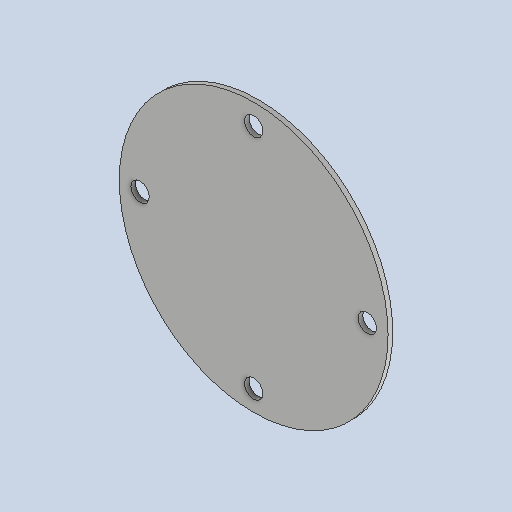
# Autodesk Inventor part: MSC 126 flange base tube
Saved by Autodesk Inventor 2025 (Build 290162010, 162A)
## iProperties
Created: 2024-07-01
Part Number: MSC 126 flange base tube
Material: Stainless Steel
Document SubType Name: Sheet Metal
Designer: pokla
Density: 8 g/cm^3
Sheet Metal Rule: AISI304 3mm Die 32
Appearance: Default
Author: pokla
Autodesk Inventor part; units mm, degrees
ref_plane "YZ Plane" through (0, 0, 0) normal (1, 0, 0) x (0, 1, 0)
ref_plane "XZ Plane" through (0, 0, 0) normal (0, 1, 0) x (-1, 0, 0)
ref_plane "XY Plane" through (0, 0, 0) normal (0, 0, 1) x (1, 0, 0)
sketch "Sketch1" plane through (0, 0, 0) normal (0, 1, 0) x (-1, 0, 0)
  circle A0 centre (0, 0) radius 87.5
  dimension "d0" = 175
  measures "d0" diameter of A0
extrude "Plate1" add sketch "Sketch1" along normal blind 3
sketch "Sketch2" plane through (0, 3, 0) normal (0, 1, 0) x (1, 0, 0)
  line L0 (-40, -40) -> (40, -40) construction
  line L1 (40, -40) -> (40, 40) construction
  line L2 (40, 40) -> (-40, 40) construction
  line L3 (-40, 40) -> (-40, -40) construction
  line L4 (40, -40) -> (-40, 40) construction
  circle A0 centre (0, 0) radius 87.5 projected
  line L5 (0, 0) -> (0, -87.5) construction
  circle A1 centre (0, -74) radius 6
  dimension "d2" = 80
  dimension "d3" = 80
  dimension "d16" = 12
  dimension "d17" = 13.5
  constraints: 12 end point, 2 parallel, 2 perpendicular, 1 centre point, 1 coincident, 1 horizontal, 1 midpoint, 1 point on line, 1 vertical alignment, 1 other
  measures "d2" distance of L2.end L1.end
  measures "d3" distance of L1.end L0.end
  measures "d16" diameter of A1
  measures "d17" distance of L5.end A1.centre
extrude "Extrusion1" cut sketch "Sketch2" against normal through all contours A1
pattern_circular "Circular Pattern1" count 4 over 360 about axis through (0, -10, 0) along (0, 1, 0) of "Extrusion1"
equation "\"d1\" = Thickness"
equation "\"BendReliefWidth\" = Thickness"
equation "\"BendReliefDepth\" = 0.5 * Thickness"
equation "\"CornerReliefSize\" = 4 * Thickness"
equation "\"MinimumRemnant\" = 2 * Thickness"
equation "\"TransitionRadius\" = BendRadius"
equation "\"JacobiRadiusSize\" = BendRadius"
equation "\"GapSize\" = Thickness"
equation "\"Thickness\" = 3"
equation "\"BendRadius\" = 5"
body "Solid1"
